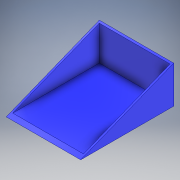
# Autodesk Inventor part: Bucket
Saved by Autodesk Inventor 2020 (Build 240168000, 168)
## iProperties
Created: 2019-10-01
Part Number: Bucket
Material: Aluminum 6061
Document SubType Name: Modeling
Designer: Matt
Mass: 157.818 g
Surface Area: 476.751 cm^2
Volume: 58.451 cm^3
Density: 2.7 g/cm^3
Appearance: Blue - Wall Paint - Glossy
Author: Matt
Autodesk Inventor part; units mm, degrees
ref_plane "YZ Plane" through (0, 0, 0) normal (1, 0, 0) x (0, 1, 0)
ref_plane "XZ Plane" through (0, 0, 0) normal (0, 1, 0) x (-1, 0, 0)
ref_plane "XY Plane" through (0, 0, 0) normal (0, 0, 1) x (1, 0, 0)
sketch "Sketch1" plane through (0, 0, 0) normal (1, 0, 0) x (0, 1, 0)
  line L0 (0, 0) -> (0, -127)
  line L1 (0, -127) -> (50.8, -127)
  line L2 (0, 0) -> (50.8, -127)
  dimension "d0" = 127
  dimension "d1" = 50.8
  constraints: 6 end point, 1 perpendicular, 1 vertical
  measures "d0" distance of L0.start L0.end
  measures "d1" distance of L0.end L1.end
extrude "Extrusion1" add sketch "Sketch1" along normal blind 101.6
shell "Shell1" thickness 2.54 removed faces 1 at (33.8667, 33.8667, -84.6667)
body "Solid1"
